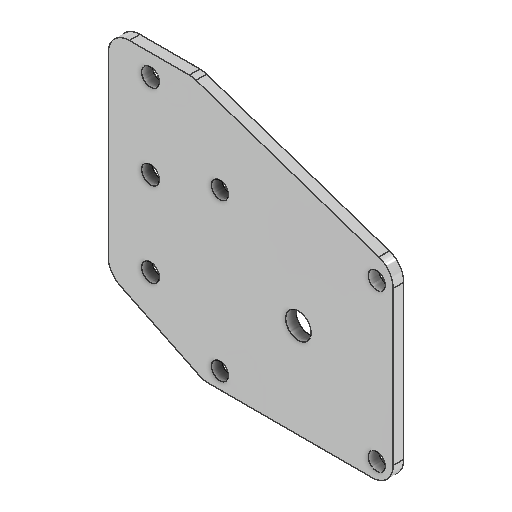
# Autodesk Inventor part: Diff Motor Bracket
Saved by Autodesk Inventor 2025.2 (Build 292293000, 293)
## iProperties
Created: 2025-02-25
Part Number: Diff Motor Bracket
Material: Generic
Document SubType Name: Modeling
Designer: Jakeg
Density: 1 g/cm^3
Appearance: Aluminum - Polished
Author: Jakeg
Autodesk Inventor part; units mm, degrees
ref_plane "YZ Plane" through (0, 0, 0) normal (1, 0, 0) x (0, 1, 0)
ref_plane "XZ Plane" through (0, 0, 0) normal (0, 1, 0) x (-1, 0, 0)
ref_plane "XY Plane" through (0, 0, 0) normal (0, 0, 1) x (1, 0, 0)
sketch "Sketch1" plane through (0, 0, 0) normal (0, 0, 1) x (1, 0, 0)
  line L0 (-39.5223, 4.2825) -> (17.4753, 4.2825)
  line L1 (17.4753, 4.2825) -> (17.4753, -52.7151)
  line L2 (17.4753, -52.7151) -> (-39.5223, -52.7151)
  line L3 (-39.5223, -52.7151) -> (-39.5223, 4.2825)
  circle A0 centre (-34.5937, -47.7865) radius 2.5527
  circle A1 centre (12.5467, -47.7865) radius 2.5527
  circle A2 centre (-34.5937, -0.6461) radius 2.5527
  circle A3 centre (12.5467, -0.6461) radius 2.5527
  line L4 (-68.1735, 24.6219) -> (-42.7735, 24.6219)
  line L5 (-42.7735, 24.6219) -> (-42.7735, -38.8781)
  line L6 (-42.7735, -38.8781) -> (-68.1735, -38.8781)
  line L7 (-68.1735, -38.8781) -> (-68.1735, 24.6219)
  circle A4 centre (-55.4735, 18.2719) radius 2.6543
  circle A5 centre (-55.4735, -32.5281) radius 2.6543
  circle A6 centre (-55.4735, -7.1281) radius 2.6543
  line L8 (-68.1735, -7.1281) -> (-42.7735, -7.1281)
  circle A7 centre (-55.4735, 46.8469) radius 8.6868
  line L9 (-42.7735, 24.6219) -> (17.4753, 4.2825)
  line L10 (-68.1735, -38.8781) -> (-39.5223, -52.7151)
  circle A8 centre (-11.0235, -24.2163) radius 3.81
  point P0 (0, 0)
  dimension "d0" = 56.9976
  dimension "d1" = 56.9976
  dimension "d3" = 5.1054
  dimension "d4" = 5.1054
  dimension "d5" = 5.1054
  dimension "d7" = 5.1054
  dimension "d15" = 28.4988
  dimension "d16" = 28.4988
  dimension "d17" = 63.5
  dimension "d18" = 25.4
  dimension "d19" = 25.4
  dimension "d20" = 0
  dimension "d21" = 5.3086
  dimension "d22" = 5.3086
  dimension "d23" = 5.3086
  dimension "d24" = 28.575
  dimension "d26" = 12.7
  dimension "d28" = 0
  dimension "d29" = 0
  dimension "d30" = 12.7
  dimension "d33" = 83.82
  dimension "d34" = 44.45
  dimension "d37" = 7.62
  dimension "d39" = 66.6666
  dimension "d40" = 66.6666
  dimension "d41" = 33.3333
  dimension "d42" = 33.3333
  constraints: 22 end point, 9 centre point, 4 parallel, 3 coincident, 3 midpoint, 2 horizontal, 2 perpendicular
  measures "d0" distance of L0.start L0.end
  measures "d1" distance of L0.end L1.end
  measures "d3" diameter of A0
  measures "d4" diameter of A1
  measures "d5" diameter of A2
  measures "d7" diameter of A3
  measures "d15" distance from line of L3 point (-11.024, -24.216)
  measures "d16" distance from line of L2 point (-11.024, -24.216)
  measures "d17" distance of L6.end L4.start
  measures "d18" distance of A6.centre A5.centre
  measures "d19" distance of A4.centre A6.centre
  measures "d20" distance from line of L8 A6.centre
  measures "d21" diameter of A4
  measures "d22" diameter of A6
  measures "d23" diameter of A5
  measures "d24" distance of A7.centre A4.centre
  measures "d26" distance from line of L7 point (-55.474, -7.128)
  measures "d28" horizontal distance of A6.centre A4.centre
  measures "d29" horizontal distance of A4.centre A7.centre
  measures "d30" distance from line of L7 A7.centre
  measures "d33" distance of point (-11.024, -24.216) A7.centre
  measures "d34" horizontal distance of point (-11.024, -24.216) A7.centre
  measures "d37" diameter of A8
  measures "d39" distance of A1.centre A2.centre
  measures "d40" distance of A3.centre A0.centre
  measures "d41" distance of A2.centre A8.centre
  measures "d42" distance of A0.centre point (-11.024, -24.216)
extrude "Extrusion1" add sketch "Sketch1" along normal blind 3.175 contours L3 L10 L6 L5 L9 L0 | L0 L1 L2 L3 | L5 L8 A6 L7 L4 | L7 L8 A6 L5 L6
fillet "Fillet1" radius 6.35 6 edges at (-42.7735, 24.6219, 1.5875) (-68.1735, 24.6219, 1.5875) (17.4753, 4.2825, 1.5875) (17.4753, -52.7151, 1.5875) (-39.5223, -52.7151, 1.5875) (-68.1735, -38.8781, 1.5875)
equation "\"d4\" = d3"
equation "\"d15\" = 0.5 * d0"
equation "\"d16\" = d15"
equation "\"d19\" = d18"
equation "\"d22\" = d21"
equation "\"d23\" = d21"
equation "\"d40\" = d39"
equation "\"d41\" = 0.5 * d39"
equation "\"d42\" = d41"
body "Solid1"
